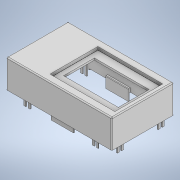
# Autodesk Inventor part: Pieza_tapa_TFM
Saved by Autodesk Inventor 2021 (Build 250183000, 183)
## iProperties
Created: 2023-07-23
Part Number: Pieza_tapa_TFM
Material: Generic
Document SubType Name: Modeling
Designer: alu01
Density: 1 g/cm^3
Appearance: Default
Author: alu01
Autodesk Inventor part; units mm, degrees
ref_plane "YZ Plane" through (0, 0, 0) normal (1, 0, 0) x (0, 1, 0)
ref_plane "XZ Plane" through (0, 0, 0) normal (0, 1, 0) x (-1, 0, 0)
ref_plane "XY Plane" through (0, 0, 0) normal (0, 0, 1) x (1, 0, 0)
sketch "Sketch2" plane through (0, 0, 0) normal (1, 0, 0) x (0, 1, 0)
  line L0 (0, 31) -> (28.5, 31)
  line L1 (28.5, 31) -> (28.5, -31)
  line L2 (28.5, -31) -> (0, -31)
  line L3 (0, -31) -> (0, 31)
  point P0 (0, 0)
  dimension "d9" = 28.5
  dimension "d10" = 62
  dimension "d11" = 31
  constraints: 8 end point, 2 parallel, 1 horizontal, 1 perpendicular
  measures "d9" distance of L0.start L0.end
  measures "d10" distance of L0.end L1.end
  measures "d11" distance from line of point (0, 0) L0
extrude "Extrusion1" add sketch "Sketch2" along normal mid plane 106
sketch "Sketch3" plane through (-53, 28.5, 31) normal (0, 1, 0) x (1, 0, 0)
  line L0 (36.85, 55.075) -> (102, 55.075)
  line L1 (102, 55.075) -> (102, 6.925)
  line L2 (102, 6.925) -> (36.85, 6.925)
  line L3 (36.85, 6.925) -> (36.85, 55.075)
  line L4 (106, 62) -> (106, 0) projected
  line L5 (0, 62) -> (106, 62) projected
  point P0 (53, 31)
  dimension "d14" = 65.15
  dimension "d15" = 48.15
  dimension "d16" = 4
  dimension "d17" = 6.925
  constraints: 8 end point, 2 parallel, 1 horizontal, 1 perpendicular
  measures "d14" distance of L0.start L0.end
  measures "d15" distance of L2.end L0.start
  measures "d16" distance between parallel lines of L4 L1
  measures "d17" distance between parallel lines of L0 L5
extrude "Extrusion2" cut sketch "Sketch3" against normal blind 3.15
sketch "Sketch4" plane through (-53, 25.35, 31) normal (0, 1, 0) x (1, 0, 0)
  circle A0 centre (38.425, 8.5) radius 1.575
  line L0 (36.85, 6.925) -> (36.85, 55.075) projected
  line L1 (102, 6.925) -> (36.85, 6.925) projected
  line L2 (69.425, 55.075) -> (69.425, 6.925)
  circle A1 centre (100.425, 8.5) radius 1.575
  line L3 (41.925, 46.5) -> (96.925, 46.5)
  line L4 (96.925, 46.5) -> (96.925, 15.5)
  line L5 (96.925, 15.5) -> (41.925, 15.5)
  line L6 (41.925, 15.5) -> (41.925, 46.5)
  line L7 (36.85, 55.075) -> (102, 55.075) projected
  line L8 (102, 55.075) -> (102, 6.925) projected
  line L9 (106, 62) -> (106, 0) projected
  line L10 (106, 31) -> (-7.1819, 31)
  point P0 (53, 31)
  dimension "d20" = 3.15
  dimension "d21" = 55
  dimension "d22" = 31
  dimension "d24" = 5.075
  dimension "d30" = 15.5
  constraints: 12 end point, 2 centre point, 2 midpoint, 2 parallel, 2 perpendicular, 2 tangent, 1 horizontal, 1 symmetric about line, 1 other
  measures "d20" diameter of A0
  measures "d21" distance of L3.start L3.end
  measures "d22" distance of L5.end L3.start
  measures "d24" distance between parallel lines of L8 L4
  measures "d30" distance from line of L3 L10.start
shell "Shell1" thickness 2 removed faces 1 at (-17.6667, 0, 10.3333)
extrude "Extrusion3" cut sketch "Sketch4" against normal blind 2 contours L10 L2 L5 L6 | L6 L3 L2 L10 | L2 L10 L4 L5 | L2 L3 L4 L10
extrude "Extrusion4" cut sketch "Sketch4" against normal blind 2 contours A0 | A1
sketch "Sketch5" plane through (-53, 0, -31) normal (0, -1, 0) x (1, 0, 0)
  line L0 (104, 54.5) -> (103, 54.5)
  line L1 (103, 54.5) -> (103, 52.5)
  line L2 (103, 52.5) -> (104, 52.5)
  line L3 (104, 52.5) -> (104, 54.5)
  line L4 (104, 50.35) -> (103, 50.35)
  line L5 (103, 50.35) -> (103, 48.35)
  line L6 (103, 48.35) -> (104, 48.35)
  line L7 (104, 48.35) -> (104, 50.35)
  line L8 (90.4, 60) -> (88.4, 60)
  line L9 (88.4, 60) -> (88.4, 59)
  line L10 (88.4, 59) -> (90.4, 59)
  line L11 (90.4, 59) -> (90.4, 60)
  line L12 (86.25, 60) -> (84.25, 60)
  line L13 (84.25, 60) -> (84.25, 59)
  line L14 (84.25, 59) -> (86.25, 59)
  line L15 (86.25, 59) -> (86.25, 60)
  line L16 (64.4855, 60) -> (41.785, 60)
  line L17 (64.4855, 58) -> (41.785, 58)
  line L18 (53, 0) -> (53, 63.4822)
  line L19 (2, 54.5) -> (3, 54.5)
  line L20 (3, 54.5) -> (3, 52.5)
  line L21 (3, 52.5) -> (2, 52.5)
  line L22 (2, 52.5) -> (2, 54.5)
  line L23 (2, 50.35) -> (3, 50.35)
  line L24 (3, 50.35) -> (3, 48.35)
  line L25 (3, 48.35) -> (2, 48.35)
  line L26 (2, 48.35) -> (2, 50.35)
  line L27 (15.6, 60) -> (17.6, 60)
  line L28 (17.6, 60) -> (17.6, 59)
  line L29 (17.6, 59) -> (15.6, 59)
  line L30 (15.6, 59) -> (15.6, 60)
  line L31 (19.75, 60) -> (21.75, 60)
  line L32 (21.75, 60) -> (21.75, 59)
  line L33 (21.75, 59) -> (19.75, 59)
  line L34 (19.75, 59) -> (19.75, 60)
  line L35 (64.4855, 58) -> (64.4855, 60)
  line L36 (41.785, 58) -> (41.785, 60)
  line L37 (0, 31) -> (143.9374, 31)
  line L38 (104, 7.5) -> (103, 7.5)
  line L39 (103, 7.5) -> (103, 9.5)
  line L40 (103, 9.5) -> (104, 9.5)
  line L41 (104, 9.5) -> (104, 7.5)
  line L42 (104, 11.65) -> (103, 11.65)
  line L43 (103, 11.65) -> (103, 13.65)
  line L44 (103, 13.65) -> (104, 13.65)
  line L45 (104, 13.65) -> (104, 11.65)
  line L46 (90.4, 2) -> (88.4, 2)
  line L47 (88.4, 2) -> (88.4, 3)
  line L48 (88.4, 3) -> (90.4, 3)
  line L49 (90.4, 3) -> (90.4, 2)
  line L50 (86.25, 2) -> (84.25, 2)
  line L51 (84.25, 2) -> (84.25, 3)
  line L52 (84.25, 3) -> (86.25, 3)
  line L53 (86.25, 3) -> (86.25, 2)
  line L54 (64.4855, 2) -> (41.785, 2)
  line L55 (64.4855, 4) -> (41.785, 4)
  line L56 (2, 7.5) -> (3, 7.5)
  line L57 (3, 7.5) -> (3, 9.5)
  line L58 (3, 9.5) -> (2, 9.5)
  line L59 (2, 9.5) -> (2, 7.5)
  line L60 (3, 11.65) -> (3, 13.65)
  line L61 (2, 11.65) -> (3, 11.65)
  line L62 (3, 13.65) -> (2, 13.65)
  line L63 (2, 13.65) -> (2, 11.65)
  line L64 (21.75, 2) -> (21.75, 3)
  line L65 (19.75, 3) -> (19.75, 2)
  line L66 (21.75, 3) -> (19.75, 3)
  line L67 (19.75, 2) -> (21.75, 2)
  line L68 (15.6, 2) -> (17.6, 2)
  line L69 (17.6, 3) -> (15.6, 3)
  line L70 (15.6, 3) -> (15.6, 2)
  line L71 (17.6, 2) -> (17.6, 3)
  line L72 (64.4855, 4) -> (64.4855, 2)
  line L73 (41.785, 4) -> (41.785, 2)
  line L74 (0, 62) -> (106, 62) projected
  line L75 (106, 62) -> (106, 0) projected
  point P0 (53, 31)
  point P1 (53, -1.4822)
  dimension "d32" = 2
  dimension "d33" = 1
  dimension "d34" = 1
  dimension "d35" = 2
  dimension "d36" = 2.15
  dimension "d37" = 2
  dimension "d38" = 1
  dimension "d40" = 2
  dimension "d41" = 1
  dimension "d42" = 2.15
  dimension "d47" = 2
  dimension "d71" = 7.5
  dimension "d72" = 15.6
  constraints: 148 end point, 53 symmetric about line, 9 parallel, 6 horizontal, 4 perpendicular, 2 vertical
  measures "d32" distance of L0.end L1.end
  measures "d33" distance of L1.end L2.end
  measures "d34" distance of L6.end L5.end
  measures "d35" distance of L4.end L5.end
  measures "d36" distance between parallel lines of L2 L4
  measures "d37" distance of L10.end L9.end
  measures "d38" distance of L10.end L8.start
  measures "d40" distance of L14.end L13.end
  measures "d41" distance of L12.end L13.end
  measures "d42" distance between parallel lines of L15 L9
  measures "d47" distance of L17.start L16.start
  measures "d71" distance between parallel lines of L0 L74
  measures "d72" distance between parallel lines of L11 L75
extrude "Extrusion5" add sketch "Sketch5" along normal blind 7 contours L3 L2 L1 L0 | L7 L6 L5 L4 | L11 L10 L9 L8 | L15 L14 L13 L12 | L19 L20 L21 L22 | L23 L24 L25 L26 | L27 L28 L29 L30 | L31 L32 L33 L34 | L38 L39 L40 L41 | L42 L43 L44 L45 | L46 L47 L48 L49 | L50 L51 L52 L53 | L59 L58 L57 L56 | L61 L63 L62 L60 | L67 L65 L66 L64 | L70 L69 L71 L68
extrude "Extrusion6" add sketch "Sketch5" against normal blind 4 contours L3 L2 L1 L0 | L7 L6 L5 L4 | L11 L10 L9 L8 | L15 L14 L13 L12 | L35 L17 L18 L16 | L18 L17 L36 L16 | L54 L73 L55 L18 | L18 L55 L72 L54 | L19 L20 L21 L22 | L23 L24 L25 L26 | L27 L28 L29 L30 | L31 L32 L33 L34 | L38 L39 L40 L41 | L42 L43 L44 L45 | L46 L47 L48 L49 | L50 L51 L52 L53 | L59 L58 L57 L56 | L61 L63 L62 L60 | L67 L65 L66 L64 | L70 L69 L71 L68
sketch "Sketch6" plane through (-53, 0, -31) normal (0, -1, 0) x (1, 0, 0)
  line L0 (41.785, 60) -> (41.785, 58) projected
  line L1 (64.4855, 60) -> (64.4855, 58) projected
  line L2 (41.785, 58) -> (64.4855, 58)
  line L3 (64.4855, 58) -> (64.4855, 58.9)
  line L4 (64.4855, 58.9) -> (41.785, 58.9)
  line L5 (41.785, 58.9) -> (41.785, 58)
  line L6 (41.785, 2) -> (41.785, 4) projected
  line L7 (64.4855, 2) -> (64.4855, 4) projected
  line L8 (41.785, 4) -> (64.4855, 4)
  line L9 (64.4855, 4) -> (64.4855, 3.1)
  line L10 (64.4855, 3.1) -> (41.785, 3.1)
  line L11 (41.785, 3.1) -> (41.785, 4)
  point P0 (53, 31)
  point P1 (41.785, 3.1)
  dimension "d53" = 0.9
  dimension "d54" = 0.9
  constraints: 16 end point, 4 parallel, 2 horizontal, 2 perpendicular, 2 point on line
  measures "d53" distance between parallel lines of L4 L2
  measures "d54" distance between parallel lines of L8 L10
extrude "Extrusion7" add sketch "Sketch6" along normal blind 7
sketch "Sketch7" plane through (-53, 0, -31) normal (0, -1, 0) x (1, 0, 0)
  line L0 (2, 7.5) -> (2, 9.5) projected
  line L1 (1, 7.5) -> (2, 7.5)
  line L2 (2, 7.5) -> (2, 9.5)
  line L3 (2, 9.5) -> (1, 9.5)
  line L4 (1, 9.5) -> (1, 7.5)
  line L5 (2, 11.65) -> (2, 13.65) projected
  line L6 (2, 11.65) -> (1, 11.65)
  line L7 (1, 11.65) -> (1, 13.65)
  line L8 (1, 13.65) -> (2, 13.65)
  line L9 (2, 13.65) -> (2, 11.65)
  line L10 (2, 48.35) -> (2, 50.35) projected
  line L11 (2, 48.35) -> (1, 48.35)
  line L12 (1, 48.35) -> (1, 50.35)
  line L13 (1, 50.35) -> (2, 50.35)
  line L14 (2, 50.35) -> (2, 48.35)
  line L15 (2, 52.5) -> (1, 52.5)
  line L16 (1, 52.5) -> (1, 54.5)
  line L17 (1, 54.5) -> (2, 54.5)
  line L18 (2, 54.5) -> (2, 52.5)
  line L19 (15.6, 60) -> (17.6, 60) projected
  line L20 (15.6, 60) -> (17.6, 60)
  line L21 (17.6, 60) -> (17.6, 61)
  line L22 (17.6, 61) -> (15.6, 61)
  line L23 (15.6, 61) -> (15.6, 60)
  line L24 (21.75, 60) -> (19.75, 60) projected
  line L25 (19.75, 60) -> (21.75, 60)
  line L26 (21.75, 60) -> (21.75, 61)
  line L27 (21.75, 61) -> (19.75, 61)
  line L28 (19.75, 61) -> (19.75, 60)
  line L29 (15.6, 2) -> (17.6, 2)
  line L30 (17.6, 2) -> (17.6, 1)
  line L31 (17.6, 1) -> (15.6, 1)
  line L32 (15.6, 1) -> (15.6, 2)
  line L33 (21.75, 2) -> (23.75, 2)
  line L34 (23.75, 2) -> (23.75, 1)
  line L35 (23.75, 1) -> (21.75, 1)
  line L36 (21.75, 1) -> (21.75, 2)
  line L37 (53, 0) -> (53, 62)
  line L38 (104, 7.5) -> (104, 9.5)
  line L39 (105, 7.5) -> (104, 7.5)
  line L40 (104, 7.5) -> (104, 9.5)
  line L41 (104, 9.5) -> (105, 9.5)
  line L42 (105, 9.5) -> (105, 7.5)
  line L43 (104, 11.65) -> (104, 13.65)
  line L44 (104, 11.65) -> (105, 11.65)
  line L45 (105, 11.65) -> (105, 13.65)
  line L46 (105, 13.65) -> (104, 13.65)
  line L47 (104, 13.65) -> (104, 11.65)
  line L48 (104, 48.35) -> (104, 50.35)
  line L49 (104, 48.35) -> (105, 48.35)
  line L50 (105, 48.35) -> (105, 50.35)
  line L51 (105, 50.35) -> (104, 50.35)
  line L52 (104, 50.35) -> (104, 48.35)
  line L53 (104, 52.5) -> (105, 52.5)
  line L54 (105, 52.5) -> (105, 54.5)
  line L55 (105, 54.5) -> (104, 54.5)
  line L56 (104, 54.5) -> (104, 52.5)
  line L57 (90.4, 60) -> (88.4, 60)
  line L58 (90.4, 60) -> (88.4, 60)
  line L59 (88.4, 60) -> (88.4, 61)
  line L60 (88.4, 61) -> (90.4, 61)
  line L61 (90.4, 61) -> (90.4, 60)
  line L62 (84.25, 60) -> (86.25, 60)
  line L63 (86.25, 60) -> (84.25, 60)
  line L64 (84.25, 60) -> (84.25, 61)
  line L65 (84.25, 61) -> (86.25, 61)
  line L66 (86.25, 61) -> (86.25, 60)
  line L67 (90.4, 2) -> (88.4, 2)
  line L68 (88.4, 2) -> (88.4, 1)
  line L69 (88.4, 1) -> (90.4, 1)
  line L70 (90.4, 1) -> (90.4, 2)
  line L71 (84.25, 2) -> (82.25, 2)
  line L72 (82.25, 2) -> (82.25, 1)
  line L73 (82.25, 1) -> (84.25, 1)
  line L74 (84.25, 1) -> (84.25, 2)
  point P0 (53, 31)
  point P1 (41.785, 58.9)
  point P2 (64.4855, 60)
  point P3 (41.785, 3.1)
  point P4 (64.4855, 2)
  point P5 (84.25, 60)
  point P6 (17.6, 60)
  dimension "d57" = 2
  dimension "d58" = 1
  dimension "d59" = 2
  dimension "d60" = 1
  dimension "d61" = 2
  dimension "d62" = 1
  constraints: 140 end point, 37 symmetric about line, 16 parallel, 8 horizontal, 8 perpendicular, 2 point on line
  measures "d57" distance of L3.end L1.start
  measures "d58" distance of L1.start L1.end
  measures "d59" distance of L22.end L21.end
  measures "d60" distance of L20.end L21.end
  measures "d61" distance of L30.end L31.end
  measures "d62" distance of L31.end L29.start
extrude "Extrusion8" add sketch "Sketch7" along normal blind 1
fillet "Fillet1" radius 0.5 54 edges at (-18.15, 26.5, 0) (-18.15, 23.35, 0) (-18.15, 24.925, -26.075) (16.425, 23.35, -26.075) (16.425, 26.5, -26.075) (-18.15, 24.925, 26.075) (16.425, 23.35, 26.075) (16.425, 26.5, 26.075) (51, 23.35, 0) (51, 24.925, -26.075) (51, 26.5, -27.5375) (51, 26.5, 27.5375) (51, 24.925, 26.075) (51, 13.25, 29) (0, 26.5, 29) (51, 13.25, -29) (0, 26.5, -29) (-51, 13.25, -29) (-51, 26.5, 0) (-51, 13.25, 29) (-36.4, 0, -30) (-36.4, -1, -30) (-30.25, 0, -30) (-30.25, -1, -30) (-36.4, -1, -29) (30.25, 0, -30) (30.25, -1, -30) (36.4, 0, -30) (36.4, -1, -30) (36.4, -1, -29) (52, 0, -22.5) (52, -1, -22.5) (51, -1, -22.5) (52, 0, -18.35) (52, -1, -18.35) (51, -1, -18.35) (52, 0, 18.35) (52, -1, 18.35) (51, -1, 18.35) (52, 0, 22.5) (52, -1, 22.5) (51, -1, 22.5) (36.4, 0, 30) (36.4, -1, 30) (36.4, -1, 29) (32.25, 0, 30) (32.25, -1, 30) (32.25, -1, 29) (-32.25, 0, 30) (-32.25, -1, 30) (-32.25, -1, 29) (-36.4, 0, 30) (-36.4, -1, 30) (-36.4, -1, 29)
fillet "Fillet2" radius 0.5 12 edges at (-52, 0, 22.5) (-52, -1, 22.5) (-51, -1, 22.5) (-52, 0, 18.35) (-52, -1, 18.35) (-51, -1, 18.35) (-52, 0, -18.35) (-52, -1, -18.35) (-51, -1, -18.35) (-52, 0, -22.5) (-52, -1, -22.5) (-51, -1, -22.5)
fillet "Fillet3" radius 0.1 2 edges at (0.1352, 0, 27.9) (0.1352, 0, -27.9)
fillet "Fillet4" radius 1 8 edges at (-53, 28.5, 0) (0, 28.5, 31) (-53, 14.25, 31) (53, 14.25, 31) (53, 28.5, 0) (0, 28.5, -31) (-53, 14.25, -31) (53, 14.25, -31)
fillet "Fillet5" radius 0.1 12 edges at (16.425, 25.35, 24.075) (-15.3625, 25.35, 24.075) (-16.15, 25.35, 23.2875) (-16.15, 25.35, -0.7875) (48.2125, 25.35, 24.075) (49, 25.35, 23.2875) (49, 25.35, -0.7875) (49, 26.925, 24.075) (-16.15, 26.925, 24.075) (-16.15, 26.925, -24.075) (16.425, 25.35, -24.075) (49, 26.925, -24.075)
fillet "Fillet6" radius 0.5 18 edges at (-36.4, 4, 28) (-32.25, 4, 28) (-50, 4, 22.5) (-50, 4, 18.35) (-50, 4, -18.35) (-50, 4, -22.5) (32.25, 4, 28) (37.4, -1.5, 28) (0.1352, 4, 27) (-36.4, 4, -28) (-32.25, 4, -28) (0.1352, 4, -27) (32.25, 4, -28) (36.4, 4, -28) (50, 4, -22.5) (50, 4, -18.35) (50, 4, 18.35) (50, 4, 22.5)
body "Solid1"
